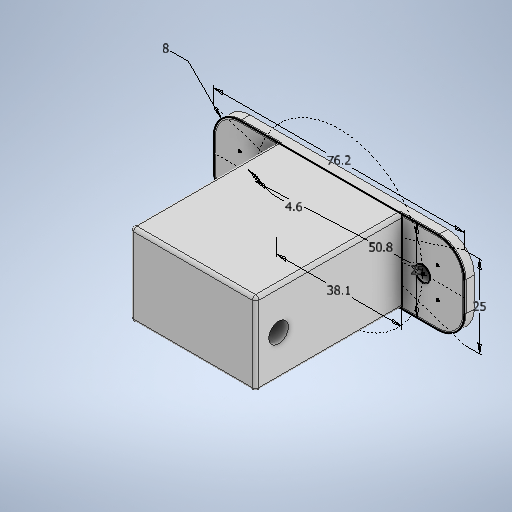
# Autodesk Inventor part: camstand1.75inch tall
Saved by Autodesk Inventor 2025 (Build 290162000, 162)
## iProperties
Created: 2025-03-15
Part Number: camstand1.75inch tall
Material: Generic
Document SubType Name: Modeling
Designer: john
Density: 1 g/cm^3
Appearance: Default
Author: john
Autodesk Inventor part; units mm, degrees
ref_plane "YZ Plane" through (0, 0, 0) normal (1, 0, 0) x (0, 1, 0)
ref_plane "XZ Plane" through (0, 0, 0) normal (0, 1, 0) x (-1, 0, 0)
ref_plane "XY Plane" through (0, 0, 0) normal (0, 0, 1) x (1, 0, 0)
sketch "Sketch1" plane through (0, 0, 0) normal (0, 0, 1) x (1, 0, 0)
  line L0 (-30.1, -12.5) -> (30.1, -12.5)
  line L1 (38.1, -4.5) -> (38.1, 4.5)
  line L2 (30.1, 12.5) -> (-30.1, 12.5)
  line L3 (-38.1, 4.5) -> (-38.1, -4.5)
  line L4 (-38.1, -12.5) -> (38.1, 12.5) construction
  line L5 (38.1, -12.5) -> (-38.1, 12.5) construction
  line L6 (-38.1, 0) -> (38.1, 0) construction
  line L7 (0, 12.5) -> (0, -12.5) construction
  circle A0 centre (0, 0) radius 25.4 construction
  line L8 (-19.05, 12.5) -> (19.05, 12.5) construction
  line L9 (19.05, 12.5) -> (19.05, -12.5)
  line L10 (19.05, -12.5) -> (-19.05, -12.5) construction
  line L11 (-19.05, -12.5) -> (-19.05, 12.5)
  line L12 (-19.05, 12.5) -> (19.05, -12.5) construction
  line L13 (19.05, 12.5) -> (-19.05, -12.5) construction
  circle A1 centre (-25.4, 0) radius 2.3
  circle A2 centre (25.4, 0) radius 2.3
  arc A3 (-30.1, 12.5) -> (-38.1, 4.5) centre (-30.1, 4.5) ccw
  arc A4 (-38.1, -4.5) -> (-30.1, -12.5) centre (-30.1, -4.5) ccw
  arc A5 (30.1, -12.5) -> (38.1, -4.5) centre (30.1, -4.5) ccw
  arc A6 (38.1, 4.5) -> (30.1, 12.5) centre (30.1, 4.5) ccw
  dimension "d2" = 50.8
  dimension "d0" = 76.2
  dimension "d1" = 25
  dimension "d3" = 38.1
  dimension "d4" = 25
  dimension "d5" = 4.6
  dimension "d6" = 8
  constraints: 28 end point, 9 point on line, 8 midpoint, 8 point on circle, 8 tangent, 6 centre point, 4 parallel, 3 equal radius, 2 horizontal, 2 perpendicular, 1 coincident, 1 horizontal alignment, 1 symmetric about line, 3 other
  measures "d0" distance of L5.end L4.end
  measures "d1" distance of L4.end L5.start
  measures "d3" distance of L9.end L10.end
  measures "d4" distance of L8.end L9.end
  measures "d5" diameter of A1
  measures "d6" radius of A3
extrude "Extrusion1" add sketch "Sketch1" against normal blind 3
extrude "Extrusion2" add sketch "Sketch1" along normal blind 44.45 contours L11 L2 L9 L0
sketch "Sketch2" plane through (19.05, -12.5, 0) normal (1, 0, 0) x (0, 0, -1)
  line L0 (-44.45, 0) -> (-44.45, 25) construction
  line L1 (-44.45, 12.5) -> (3, 12.5) construction
  line L2 (3, 8) -> (3, 17) construction
  circle A0 centre (-37.45, 12.5) radius 3
  point P0 (0, 12.5)
  dimension "d11" = 6
  dimension "d12" = 7
  constraints: 2 end point, 2 midpoint, 1 centre point, 1 point on line
  measures "d11" diameter of A0
  measures "d12" distance from line of A0.centre L0
extrude "Extrusion3" cut sketch "Sketch2" against normal blind 44.45
fillet "Fillet1" radius 1 4 edges at (19.05, -12.5, 22.225) (19.05, 12.5, 22.225) (-19.05, 12.5, 22.225) (-19.05, -12.5, 22.225)
fillet "Fillet2" radius 1 8 edges at (-18.7571, -12.2071, 44.45) (0, -12.5, 44.45) (18.7571, -12.2071, 44.45) (19.05, 0, 44.45) (18.7571, 12.2071, 44.45) (0, 12.5, 44.45) (-18.7571, 12.2071, 44.45) (-19.05, 0, 44.45)
fillet "Fillet3" radius 0.5 14 edges at (-35.7569, -10.1569, 0) (-18.55, -12.5, 0) (-24.575, -12.5, 0) (-35.7569, 10.1569, 0) (-18.55, 12.5, 0) (-24.575, 12.5, 0) (-38.1, 0, 0) (38.1, 0, 0) (35.7569, 10.1569, 0) (18.55, 12.5, 0) (24.575, 12.5, 0) (18.55, -12.5, 0) (24.575, -12.5, 0) (35.7569, -10.1569, 0)
body "Solid1"
